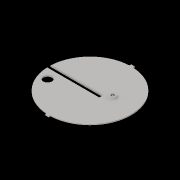
# Autodesk Inventor part: LUXCAN TAPA LISA
Saved by Autodesk Inventor 2016 (Build 200138000, 138)
## iProperties
Created: 2018-08-10
Part Number: LUXCAN TAPA LISA
Material: Generic
Document SubType Name: Sheet Metal
Designer: jocdurso
Density: 1 g/cm^3
Sheet Metal Rule: Default
Appearance: Default
Author: jocdurso
Autodesk Inventor part; units mm, degrees
ref_plane "XZ Plane" through (0, 0, 0) normal (0, 1, 0) x (-1, 0, 0)
ref_plane "XY Plane" through (0, 0, 0) normal (0, 0, 1) x (1, 0, 0)
sketch "Sketch1" plane through (0, 0, 0) normal (0, 1, 0) x (-1, 0, 0)
  circle A0 centre (0, 0) radius 48.5
  dimension "d0" = 97
  measures "d0" diameter of A0
extrude "Plate1" add sketch "Sketch1" along normal blind 1.2
sketch "Sketch2" plane through (0, 0, 0) normal (0, 1, 0) x (-1, 0, 0)
  circle A0 centre (-20.1, -6.7) radius 2
  point P0 (0, 0)
  dimension "d2" = 4
  dimension "d3" = 20.1
  dimension "d4" = 6.7
  constraints: 1 centre point, 1 coincident
  measures "d2" diameter of A0
  measures "d3" horizontal distance of point (0, 0) point (-20.1, -6.7)
  measures "d4" vertical distance of point (-20.1, -6.7) point (0, 0)
hole "Hole1" at (20.1, 0, -6.7) direction (0, 1, 0) diameter 7.6 end through all
sketch "Sketch3" plane through (0, 1.2, 0) normal (0, 1, 0) x (1, 0, 0)
  point P0 (0, 0)
  point P1 (-36.5, -13.5)
  dimension "d12" = 13.5
  dimension "d13" = 36.5
  measures "d12" vertical distance of point (0, 0) point (-36.5, -13.5)
  measures "d13" horizontal distance of point (0, 0) point (-36.5, -13.5)
hole "Hole2" at (-36.5, 1.2, 13.5) direction (0, -1, 0) diameter 10.5 end through all
sketch "Sketch5" plane through (0, 1.2, 0) normal (0, 1, 0) x (1, 0, 0)
  line L0 (-2, 50.65) -> (2, 50.65)
  line L1 (2, 50.65) -> (2, -50.65)
  line L2 (2, -50.65) -> (-2, -50.65)
  line L3 (-2, -50.65) -> (-2, 50.65)
  circle A0 centre (0, 0) radius 51
  point P0 (0, 50.65)
  point P1 (2, 0)
  dimension "d26" = 4
  dimension "d27" = 101.3
  dimension "d33" = 102
  measures "d26" distance of L0.start L0.end
  measures "d27" distance of L2.end L0.start
  measures "d33" diameter of A0
sheet face with bend "Face2" sketch "Sketch5" thickness 1.2 toward (0, -1, 0) bend radius 1.2 relief straight relief width 1.2 relief depth 0.6 contours L0 L1 L2 L3
bend "Bend1"
sketch "Sketch4" plane through (0, 1.2, 0) normal (0, 1, 0) x (1, 0, 0)
  line L0 (-67, 2) -> (13, 2)
  line L1 (13, 2) -> (13, -2)
  line L2 (13, -2) -> (-67, -2)
  line L3 (-67, -2) -> (-67, 2)
  point P0 (0, 0)
  point P1 (13, 0)
  dimension "d21" = 4
  dimension "d22" = 80
  dimension "d23" = 13
  constraints: 8 end point, 2 parallel, 1 horizontal, 1 horizontal alignment, 1 midpoint, 1 perpendicular
  measures "d21" distance of L2.end L0.start
  measures "d22" distance of L0.start L0.end
  measures "d23" distance from line of L1 point (0, 0)
extrude "Cut1" cut sketch "Sketch4" against normal blind 1.2
ref_plane "Work Plane1" through (20.1, 1.2, -6.7) normal (1, 0, 0) x (0, 1, 0)
sketch "Sketch6" plane through (0, 1.2, 0) normal (0, 1, 0) x (1, 0, 0)
  circle A0 centre (20.1, 6.7) radius 3.8 projected
  circle A1 centre (20.1, 6.7) radius 3.8
  circle A2 centre (20.1, 6.7) radius 5
  point P0 (0, 0)
  dimension "d34" = 1.2
  constraints: 2 centre point, 2 coincident, 1 concentric
  measures "d34" radial gap between concentric circles of A2 A0
ref_plane "Work Plane2" through (0, 3, 0) normal (0, 1, 0) x (1, 0, 0)
sketch "Sketch7" plane through (0, 3, 0) normal (0, 1, 0) x (1, 0, 0)
  circle A0 centre (20.1, 6.7) radius 2
  circle A1 centre (20.1, 6.7) radius 3.2
  point P0 (0, 0)
  dimension "d36" = 4
  dimension "d37" = 1.2
  constraints: 2 centre point, 1 coincident
  measures "d36" diameter of A0
  measures "d37" radial gap between concentric circles of A0 A1
sketch "Sketch8" plane through (20.1, 1.2, -6.7) normal (1, 0, 0) x (0, 1, 0)
  line L0 (0, 0) -> (1.7904, 0)
  point P0 (-1.2, 6.7)
  constraints: 2 end point, 1 horizontal
sketch "Sketch9" plane through (20.1, 1.2, -6.7) normal (1, 0, 0) x (0, 1, 0)
  line L0 (1.8, -3.2) -> (1.8, 3.2) projected
  line L1 (0, -5) -> (0, 5) projected
  line L2 (0, 3.8) -> (0, -3.8) projected
  line L3 (0, 3.8) -> (1.8, 2)
  line L4 (1.8, 2) -> (1.8, 3.2)
  line L5 (1.8, 3.2) -> (0, 5)
  line L6 (0, 5) -> (0, 3.8)
  line L7 (-1.8, 0) -> (2.4, 0) projected
  point P0 (-1.2, 6.7)
  constraints: 8 end point, 2 collinear, 1 parallel, 1 point on line
revolve "Revolution1" add sketch "Sketch9" angle 360 about axis through (20.1, 0, -6.7) along (0, 1, 0) contours L3 L1 L5 L0
equation "\"d10\" = Thickness"
equation "\"d19\" = Thickness"
equation "\"d24\" = Thickness"
equation "\"d28\" = BendRadius"
equation "\"d29\" = BendReliefWidth"
equation "\"d31\" = MinimumRemnant"
equation "\"d30\" = BendReliefDepth"
equation "\"d32\" = BendRadius"
equation "\"BendRadius\" = Thickness"
equation "\"BendReliefWidth\" = Thickness"
equation "\"BendReliefDepth\" = 0.5 * Thickness"
equation "\"CornerReliefSize\" = 4 * Thickness"
equation "\"MinimumRemnant\" = 2 * Thickness"
equation "\"TransitionRadius\" = BendRadius"
equation "\"JacobiRadiusSize\" = BendRadius"
equation "\"GapSize\" = Thickness"
equation "\"d1\" = BendRadius"
equation "\"Thickness\" = 1.2"
body "Solid1"
